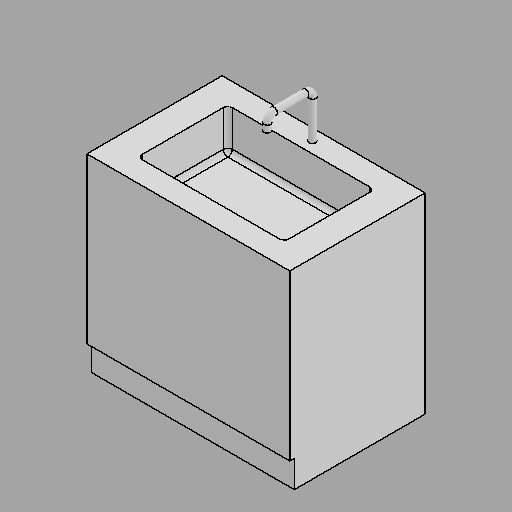
# Autodesk Inventor part: Mobile lavandino
Saved by Autodesk Inventor 2025.2 (Build 292293000, 293)
## iProperties
Created: 2025-08-13
Part Number: Mobile lavandino
Material: Generic
Document SubType Name: Modeling
Designer: Luca
Density: 1 g/cm^3
Appearance: Default
Mass: 275541 g
Surface Area: 30619.3 cm^2
Volume: 275541 cm^3
Author: Luca
Autodesk Inventor part; units mm, degrees
ref_plane "YZ Plane" through (0, 0, 0) normal (1, 0, 0) x (0, 1, 0)
ref_plane "XZ Plane" through (0, 0, 0) normal (0, 1, 0) x (-1, 0, 0)
ref_plane "XY Plane" through (0, 0, 0) normal (0, 0, 1) x (1, 0, 0)
sketch "Sketch1" plane through (0, 0, 0) normal (0, 1, 0) x (-1, 0, 0)
  line L0 (450, 0) -> (-450, 0)
  line L1 (-450, 0) -> (-450, 600)
  line L2 (-450, 600) -> (450, 600)
  line L3 (450, 600) -> (450, 0)
  point P0 (0, 0)
  point P1 (0, 0)
  dimension "d0" = 900
  dimension "d1" = 600
  constraints: 8 end point, 2 parallel, 1 coincident, 1 horizontal, 1 midpoint, 1 perpendicular
  measures "d0" distance of L1.end L2.end
  measures "d1" distance of L0.end L1.end
extrude "Extrusion1" add sketch "Sketch1" along normal blind 850
sketch "Sketch2" plane through (0, 850, 0) normal (0, 1, 0) x (1, 0, 0)
  line L0 (-325, -500) -> (325, -500)
  line L1 (325, -500) -> (325, -100)
  line L2 (325, -100) -> (-325, -100)
  line L3 (-325, -100) -> (-325, -500)
  line L4 (-325, -500) -> (325, -100) construction
  line L5 (325, -500) -> (-325, -100) construction
  line L6 (-450, 0) -> (-450, -600) projected
  line L7 (-450, -600) -> (450, -600) projected
  point P0 (0, 0)
  point P1 (0, -300)
  point P2 (-450, -300)
  point P3 (-450, -300)
  point P4 (0, -600)
  dimension "d4" = 650
  dimension "d5" = 400
  constraints: 12 end point, 5 midpoint, 2 parallel, 1 horizontal, 1 horizontal alignment, 1 perpendicular, 1 vertical alignment
  measures "d4" distance of L2.end L1.end
  measures "d5" distance of L1.end L0.end
extrude "Extrusion2" cut sketch "Sketch2" against normal blind 180
fillet "Fillet1" radius 20 8 edges at (-325, 760, 100) (-325, 670, 300) (0, 670, 100) (-325, 760, 500) (0, 670, 500) (325, 670, 300) (325, 760, 500) (325, 760, 100)
sketch "Sketch3" plane through (-450, 0, 600) normal (0, 0, 1) x (1, 0, 0)
  line L0 (0, 0) -> (900, 0) projected
  line L1 (900, 0) -> (900, 850) projected
  line L2 (0, 0) -> (900, 0)
  line L3 (900, 0) -> (900, 120)
  line L4 (900, 120) -> (0, 120)
  line L5 (0, 120) -> (0, 0)
  point P0 (450, 0)
  dimension "d9" = 120
  constraints: 8 end point, 2 parallel, 1 horizontal, 1 perpendicular, 1 point on line
  measures "d9" distance of L3.end L2.end
extrude "Extrusion3" cut sketch "Sketch3" against normal blind 20
sketch "Sketch4" plane through (0, 0, 0) normal (1, 0, 0) x (0, 1, 0)
  line L0 (850, 50) -> (1020, 50)
  arc A0 (1020, 50) -> (1050, 80) centre (1020, 80) ccw
  line L1 (1050, 80) -> (1050, 220)
  arc A1 (1050, 220) -> (1020, 250) centre (1020, 220) ccw
  line L2 (1020, 250) -> (990, 250)
  line L3 (850, 600) -> (850, 0) projected
  line L4 (850, 0) -> (850, 600) projected
  line L5 (850, 120) -> (850, 100) projected
  line L6 (850, 120) -> (850, 480) projected
  line L7 (850, 500) -> (850, 480) projected
  line L8 (850, 480) -> (850, 500) projected
  line L9 (850, 480) -> (850, 120) projected
  line L10 (850, 100) -> (850, 120) projected
  point P0 (0, 0)
  dimension "d12" = 60
  dimension "d13" = 200
  dimension "d14" = 50
  dimension "d16" = 30
  constraints: 6 end point, 4 point on circle, 4 tangent, 2 centre point, 2 perpendicular, 1 equal radius
  measures "d12" distance from line of L2.end L1
  measures "d13" distance between parallel lines of L0 L2
  measures "d14" distance from line of L3.end L0
  measures "d16" radius of A0
sketch "Sketch5" plane through (0, 850, 0) normal (0, 1, 0) x (1, 0, 0)
  circle A0 centre (0, -50) radius 15
  point P0 (0, 0)
  dimension "d17" = 30
  constraints: 1 centre point, 1 coincident
  measures "d17" diameter of A0
sweep "Sweep1" add profiles "Sketch5" path "Sketch4" path curves L0 A0 L1 A1 L2
body "Solid1"
